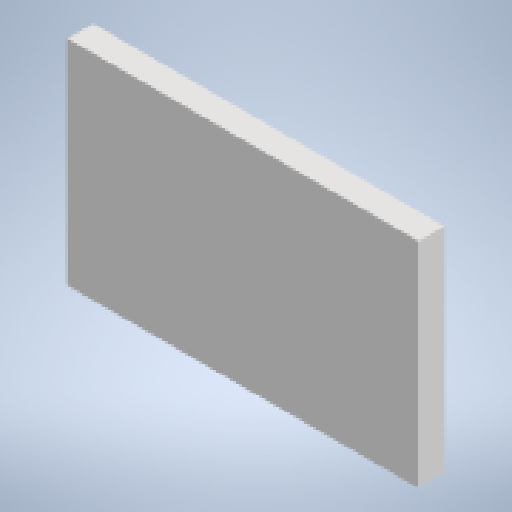
# Autodesk Inventor part: battery_5000
Saved by Autodesk Inventor 2025.2 (Build 292293000, 293)
## iProperties
Created: 2025-05-31
Part Number: battery_5000
Material: Generisch
Document SubType Name: Modeling
Designer: Jansc
Density: 1 g/cm^3
Appearance: Vorgabe
Author: Jansc
Autodesk Inventor part; units mm, degrees
ref_plane "YZ Plane" through (0, 0, 0) normal (1, 0, 0) x (0, 1, 0)
ref_plane "XZ Plane" through (0, 0, 0) normal (0, 1, 0) x (-1, 0, 0)
ref_plane "XY Plane" through (0, 0, 0) normal (0, 0, 1) x (1, 0, 0)
sketch "Skizze1" plane through (0, 0, 0) normal (0, 1, 0) x (-1, 0, 0)
  line L0 (-95.0798, 0) -> (-13.0798, 0)
  line L1 (-13.0798, 0) -> (-13.0798, -50)
  line L2 (-13.0798, -50) -> (-95.0798, -50)
  line L3 (-95.0798, -50) -> (-95.0798, 0)
  point P0 (0, 0)
  dimension "d0" = 82
  dimension "d1" = 50
  constraints: 8 end point, 2 parallel, 1 horizontal, 1 perpendicular
  measures "d0" distance of L1.end L2.end
  measures "d1" distance of L0.end L1.end
extrude "Extrusion1" add sketch "Skizze1" along normal blind 6
